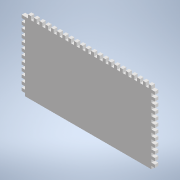
# Autodesk Inventor part: long
Saved by Autodesk Inventor 2022 (Build 260153000, 153)
## iProperties
Created: 2023-05-26
Part Number: long
Material: Типовые
Document SubType Name: Modeling
Designer: korsh624
Density: 1 g/cm^3
Appearance: По умолчанию
Author: korsh624
Autodesk Inventor part; units mm, degrees
ref_plane "YZ Plane" through (0, 0, 0) normal (1, 0, 0) x (0, 1, 0)
ref_plane "XZ Plane" through (0, 0, 0) normal (0, 1, 0) x (-1, 0, 0)
ref_plane "XY Plane" through (0, 0, 0) normal (0, 0, 1) x (1, 0, 0)
sketch "Эскиз1" plane through (0, 0, 0) normal (0, 0, 1) x (1, 0, 0)
  line L0 (0, 0) -> (5, 0) projected
  line L1 (5, 0) -> (5, 6) projected
  line L2 (0, 6) -> (5, 6) projected
  line L3 (0, 0) -> (0, 6) projected
  line L4 (-5, 0) -> (0, 0) projected
  line L5 (10, 0) -> (15, 0) projected
  line L6 (15, 0) -> (15, 6) projected
  line L7 (10, 6) -> (15, 6) projected
  line L8 (10, 0) -> (10, 6) projected
  line L9 (20, 0) -> (25, 0) projected
  line L10 (25, 0) -> (25, 6) projected
  line L11 (20, 6) -> (25, 6) projected
  line L12 (20, 0) -> (20, 6) projected
  line L13 (30, 0) -> (35, 0) projected
  line L14 (35, 0) -> (35, 6) projected
  line L15 (30, 6) -> (35, 6) projected
  line L16 (30, 0) -> (30, 6) projected
  line L17 (40, 0) -> (45, 0) projected
  line L18 (45, 0) -> (45, 6) projected
  line L19 (40, 6) -> (45, 6) projected
  line L20 (40, 0) -> (40, 6) projected
  line L21 (50, 0) -> (55, 0) projected
  line L22 (55, 0) -> (55, 6) projected
  line L23 (50, 6) -> (55, 6) projected
  line L24 (50, 0) -> (50, 6) projected
  line L25 (60, 0) -> (65, 0) projected
  line L26 (65, 0) -> (65, 6) projected
  line L27 (60, 6) -> (65, 6) projected
  line L28 (60, 0) -> (60, 6) projected
  line L29 (70, 0) -> (75, 0) projected
  line L30 (75, 0) -> (75, 6) projected
  line L31 (70, 6) -> (75, 6) projected
  line L32 (70, 0) -> (70, 6) projected
  line L33 (80, 0) -> (85, 0) projected
  line L34 (85, 0) -> (85, 6) projected
  line L35 (80, 6) -> (85, 6) projected
  line L36 (80, 0) -> (80, 6) projected
  line L37 (90, 0) -> (95, 0) projected
  line L38 (95, 0) -> (95, 6) projected
  line L39 (90, 6) -> (95, 6) projected
  line L40 (90, 0) -> (90, 6) projected
  line L41 (100, 0) -> (105, 0) projected
  line L42 (105, 0) -> (105, 6) projected
  line L43 (100, 6) -> (105, 6) projected
  line L44 (100, 0) -> (100, 6) projected
  line L45 (110, 0) -> (115, 0) projected
  line L46 (115, 0) -> (115, 6) projected
  line L47 (110, 6) -> (115, 6) projected
  line L48 (110, 0) -> (110, 6) projected
  line L49 (120, 0) -> (125, 0) projected
  line L50 (125, 0) -> (125, 6) projected
  line L51 (120, 6) -> (125, 6) projected
  line L52 (120, 0) -> (120, 6) projected
  line L53 (130, 0) -> (135, 0) projected
  line L54 (135, 0) -> (135, 6) projected
  line L55 (130, 6) -> (135, 6) projected
  line L56 (130, 0) -> (130, 6) projected
  line L57 (140, 0) -> (145, 0) projected
  line L58 (145, 0) -> (145, 6) projected
  line L59 (140, 6) -> (145, 6) projected
  line L60 (140, 0) -> (140, 6) projected
  line L61 (150, 0) -> (155, 0) projected
  line L62 (155, 0) -> (155, 6) projected
  line L63 (150, 6) -> (155, 6) projected
  line L64 (150, 0) -> (150, 6) projected
  line L65 (165, 0) -> (165, 6) projected
  line L66 (160, 0) -> (165, 0) projected
  line L67 (165, 0) -> (165, 6) projected
  line L68 (160, 6) -> (165, 6) projected
  line L69 (160, 0) -> (160, 6) projected
  line L70 (170, 0) -> (175, 0) projected
  line L71 (175, 0) -> (175, 6) projected
  line L72 (170, 6) -> (175, 6) projected
  line L73 (170, 0) -> (170, 6) projected
  line L74 (180, 0) -> (185, 0) projected
  line L75 (185, 0) -> (185, 6) projected
  line L76 (180, 6) -> (185, 6) projected
  line L77 (180, 0) -> (180, 6) projected
  line L78 (190, 0) -> (195, 0) projected
  line L79 (195, 0) -> (195, 6) projected
  line L80 (190, 6) -> (195, 6) projected
  line L81 (190, 0) -> (190, 6) projected
  line L82 (200, 0) -> (205, 0) projected
  line L83 (205, 0) -> (205, 6) projected
  line L84 (200, 6) -> (205, 6) projected
  line L85 (200, 0) -> (200, 6) projected
  line L86 (210, 0) -> (221, 0) projected
  line L87 (205, 0) -> (210, 0) projected
  line L88 (215, 0) -> (215, 6) projected
  line L89 (-5, 0) -> (215, 0)
  line L90 (215, 0) -> (215, -120)
  line L91 (215, -120) -> (-5, -120)
  line L92 (-5, -120) -> (-5, 0)
  line L93 (215, 0) -> (210, 0)
  line L94 (210, 0) -> (210, 6)
  line L95 (210, 6) -> (215, 6)
  line L96 (215, 6) -> (215, 0)
  line L97 (-5, 0) -> (-11, 0)
  line L98 (-11, 0) -> (-11, -5)
  line L99 (-11, -5) -> (-5, -5)
  line L100 (-5, -5) -> (-5, 0)
  line L101 (-5, -10) -> (-11, -10)
  line L102 (-11, -10) -> (-11, -15)
  line L103 (-11, -15) -> (-5, -15)
  line L104 (-5, -15) -> (-5, -10)
  line L105 (-5, -20) -> (-11, -20)
  line L106 (-11, -20) -> (-11, -25)
  line L107 (-11, -25) -> (-5, -25)
  line L108 (-5, -25) -> (-5, -20)
  line L109 (-5, -30) -> (-11, -30)
  line L110 (-11, -30) -> (-11, -35)
  line L111 (-11, -35) -> (-5, -35)
  line L112 (-5, -35) -> (-5, -30)
  line L113 (-5, -40) -> (-11, -40)
  line L114 (-11, -40) -> (-11, -45)
  line L115 (-11, -45) -> (-5, -45)
  line L116 (-5, -45) -> (-5, -40)
  line L117 (-5, -50) -> (-11, -50)
  line L118 (-11, -50) -> (-11, -55)
  line L119 (-11, -55) -> (-5, -55)
  line L120 (-5, -55) -> (-5, -50)
  line L121 (-5, -60) -> (-11, -60)
  line L122 (-11, -60) -> (-11, -65)
  line L123 (-11, -65) -> (-5, -65)
  line L124 (-5, -65) -> (-5, -60)
  line L125 (-5, -70) -> (-11, -70)
  line L126 (-11, -70) -> (-11, -75)
  line L127 (-11, -75) -> (-5, -75)
  line L128 (-5, -75) -> (-5, -70)
  line L129 (-5, -80) -> (-11, -80)
  line L130 (-11, -80) -> (-11, -85)
  line L131 (-11, -85) -> (-5, -85)
  line L132 (-5, -85) -> (-5, -80)
  line L133 (-5, -90) -> (-11, -90)
  line L134 (-11, -90) -> (-11, -95)
  line L135 (-11, -95) -> (-5, -95)
  line L136 (-5, -95) -> (-5, -90)
  line L137 (-5, -100) -> (-11, -100)
  line L138 (-11, -100) -> (-11, -105)
  line L139 (-11, -105) -> (-5, -105)
  line L140 (-5, -105) -> (-5, -100)
  line L141 (-5, -110) -> (-11, -110)
  line L142 (-11, -110) -> (-11, -115)
  line L143 (-11, -115) -> (-5, -115)
  line L144 (-5, -115) -> (-5, -110)
  line L145 (215, 0) -> (221, 0)
  line L146 (221, 0) -> (221, -5)
  line L147 (221, -5) -> (215, -5)
  line L148 (215, -5) -> (215, 0)
  line L149 (215, -15) -> (215, -10)
  line L150 (215, -10) -> (221, -10)
  line L151 (221, -10) -> (221, -15)
  line L152 (221, -15) -> (215, -15)
  line L153 (215, -25) -> (215, -20)
  line L154 (215, -20) -> (221, -20)
  line L155 (221, -20) -> (221, -25)
  line L156 (221, -25) -> (215, -25)
  line L157 (215, -35) -> (215, -30)
  line L158 (215, -30) -> (221, -30)
  line L159 (221, -30) -> (221, -35)
  line L160 (221, -35) -> (215, -35)
  line L161 (215, -45) -> (215, -40)
  line L162 (215, -40) -> (221, -40)
  line L163 (221, -40) -> (221, -45)
  line L164 (221, -45) -> (215, -45)
  line L165 (215, -55) -> (215, -50)
  line L166 (215, -50) -> (221, -50)
  line L167 (221, -50) -> (221, -55)
  line L168 (221, -55) -> (215, -55)
  line L169 (215, -65) -> (215, -60)
  line L170 (215, -60) -> (221, -60)
  line L171 (221, -60) -> (221, -65)
  line L172 (221, -65) -> (215, -65)
  line L173 (215, -75) -> (215, -70)
  line L174 (215, -70) -> (221, -70)
  line L175 (221, -70) -> (221, -75)
  line L176 (221, -75) -> (215, -75)
  line L177 (215, -85) -> (215, -80)
  line L178 (215, -80) -> (221, -80)
  line L179 (221, -80) -> (221, -85)
  line L180 (221, -85) -> (215, -85)
  line L181 (215, -95) -> (215, -90)
  line L182 (215, -90) -> (221, -90)
  line L183 (221, -90) -> (221, -95)
  line L184 (221, -95) -> (215, -95)
  line L185 (215, -105) -> (215, -100)
  line L186 (215, -100) -> (221, -100)
  line L187 (221, -100) -> (221, -105)
  line L188 (221, -105) -> (215, -105)
  line L189 (215, -115) -> (215, -110)
  line L190 (215, -110) -> (221, -110)
  line L191 (221, -110) -> (221, -115)
  line L192 (221, -115) -> (215, -115)
  dimension "d0" = 120
  dimension "d1" = 6
  dimension "d2" = 5
  dimension "d5" = 10
  dimension "d10" = 5
  dimension "d13" = 10
  constraints: 202 end point, 88 vertical alignment, 50 parallel, 44 collinear, 4 horizontal, 3 perpendicular, 9 other
  measures "d0" distance of L91.end L4.start
  measures "d1" distance of L99.end L98.end
  measures "d2" distance of L98.end L97.end
  measures "d5" distance of L97.end L101.end
  measures "d10" distance of L145.end L146.end
  measures "d13" distance of L93.start L149.end
extrude "Выдавливание1" add sketch "Эскиз1" along normal blind 6
